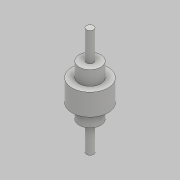
# Autodesk Inventor part: exercise1-1
Saved by Autodesk Inventor 2018 (Build 220112000, 112)
## iProperties
Created: 2020-09-19
Part Number: exercise1-1
Material: 一般
Document SubType Name: Modeling
Designer: 王鼎鈞
Density: 1 g/cm^3
Appearance: 預設
Author: 王鼎鈞
Autodesk Inventor part; units mm, degrees
ref_plane "YZ Plane" through (0, 0, 0) normal (1, 0, 0) x (0, 1, 0)
ref_plane "XZ Plane" through (0, 0, 0) normal (0, 1, 0) x (-1, 0, 0)
ref_plane "XY Plane" through (0, 0, 0) normal (0, 0, 1) x (1, 0, 0)
sketch "草圖1" plane through (0, 0, 0) normal (1, 0, 0) x (0, 1, 0)
  line L0 (-10, 0) -> (60, 0) projected
  line L1 (0, -60) -> (0, 360) projected
  line L2 (0, 0) -> (10, 0)
  line L3 (10, 0) -> (10, 300)
  line L4 (10, 300) -> (0, 300)
  line L5 (0, 300) -> (0, 0)
  line L6 (0, 80) -> (30, 80)
  line L7 (30, 80) -> (30, 120)
  line L8 (30, 120) -> (0, 120)
  line L9 (0, 120) -> (0, 80)
  line L10 (0, 120) -> (50, 120)
  line L11 (50, 120) -> (50, 180)
  line L12 (50, 180) -> (0, 180)
  line L13 (0, 180) -> (0, 120)
  line L14 (0, 180) -> (39.1578, 180)
  line L15 (0, 209.2593) -> (0, 180)
  line L16 (0, 180) -> (30, 180)
  line L17 (30, 180) -> (30, 220)
  line L18 (30, 220) -> (0, 220)
  line L19 (0, 220) -> (0, 180)
  dimension "d0" = 10
  dimension "d1" = 300
  dimension "d2" = 80
  dimension "d3" = 40
  dimension "d4" = 30
  dimension "d5" = 0
  dimension "d6" = 80
  dimension "d9" = 40
  dimension "d10" = 0
  dimension "d11" = 50
  dimension "d12" = 30
  constraints: 36 end point, 8 parallel, 5 horizontal, 4 perpendicular, 1 point on line
  measures "d0" distance of L4.end L3.end
  measures "d1" distance of L3.end L2.end
  measures "d2" distance between parallel lines of L0 L6
  measures "d3" distance of L6.end L7.end
  measures "d4" distance of L6.start L6.end
  measures "d5" distance between parallel lines of L5 L19
  measures "d6" distance between parallel lines of L4 L18
  measures "d9" distance of L16.end L17.end
  measures "d10" distance between parallel lines of L14 L16
  measures "d11" distance of L11.end L12.end
  measures "d12" distance of L17.end L18.end
revolve "迴轉1" add sketch "草圖1" angle 360 about axis through (0, 0, 300) along (0, 0, -1)
